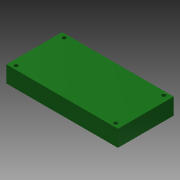
# Autodesk Inventor part: electronics
Saved by Autodesk Inventor 2013 (Build 170138000, 138)
## iProperties
Created: 2013-07-26
Part Number: electronics
Material: Generic
Document SubType Name: Modeling
Designer: employee
Density: 1 g/cm^3
Mass: 25.6248 g
Surface Area: 119.876 cm^2
Volume: 25.6248 cm^3
Author: employee
Autodesk Inventor part; units mm, degrees
ref_plane "YZ Plane" through (0, 0, 0) normal (1, 0, 0) x (0, 1, 0)
ref_plane "XZ Plane" through (0, 0, 0) normal (0, 1, 0) x (-1, 0, 0)
ref_plane "XY Plane" through (0, 0, 0) normal (0, 0, 1) x (1, 0, 0)
sketch "Sketch1" plane through (0, 0, 0) normal (0, 0, 1) x (1, 0, 0)
  line L0 (-50.8, -25.4) -> (50.8, -25.4)
  line L1 (50.8, -25.4) -> (50.8, 25.4)
  line L2 (50.8, 25.4) -> (-50.8, 25.4)
  line L3 (-50.8, 25.4) -> (-50.8, -25.4)
  point P0 (0, 0)
  point P1 (0, 25.4)
  point P2 (50.8, 0)
  dimension "d10" = 6.5
  dimension "d0" = 50.8
  dimension "d2" = 101.6
  constraints: 8 end point, 2 midpoint, 2 parallel, 1 horizontal, 1 horizontal alignment, 1 perpendicular, 1 vertical alignment
  measures "d0" distance of L0.end L1.end
  measures "d2" distance of L0.start L0.end
extrude "Extrusion1" add sketch "Sketch1" along normal blind 15
sketch "Sketch2" plane through (0, 0, 15) normal (0, 0, 1) x (1, 0, 0)
  line L0 (50.8, -25.4) -> (50.8, 25.4) projected
  line L1 (50.8, 25.4) -> (-50.8, 25.4) projected
  line L2 (-45.339, 21.9075) -> (45.339, 21.9075)
  line L3 (45.339, 21.9075) -> (45.339, -21.9075)
  line L4 (45.339, -21.9075) -> (-45.339, -21.9075)
  line L5 (-45.339, -21.9075) -> (-45.339, 21.9075)
  point P0 (45.339, 0)
  point P1 (50.8, 0)
  point P2 (0, 21.9075)
  point P3 (0, 25.4)
  dimension "d5" = 43.815
  dimension "d7" = 90.678
  constraints: 8 end point, 4 midpoint, 2 parallel, 1 horizontal, 1 horizontal alignment, 1 perpendicular, 1 vertical alignment
  measures "d5" distance of L2.end L3.end
  measures "d7" distance of L2.start L2.end
hole "Hole1" at (-45.339, 21.9075, 15) at (45.339, 21.9075, 15) at (45.339, -21.9075, 15) at (-45.339, -21.9075, 15) direction (0, 0, -1) diameter 3.4 end through all clearance for "Socket Head Cap Screw" size "M3" standard "Ansi Metric M Profile"
sketch "Sketch3" plane through (-50.8, -25.4, 0) normal (-1, 0, 0) x (0, 0, 1)
  line L0 (0, 50.8) -> (0, 0) projected
  line L1 (0, 0) -> (15, 0) projected
  circle A0 centre (6, 14.9) radius 5
  point P0 (0, 25.4)
  dimension "d15" = 6
  dimension "d16" = 14.9
  dimension "d17" = 10
  constraints: 1 centre point
  measures "d15" distance from line of A0.centre L0
  measures "d16" distance from line of A0.centre L1
  measures "d17" diameter of A0
extrude "Extrusion2" add sketch "Sketch3" along normal blind 10
sketch "Sketch4" plane through (-50.8, 25.4, 0) normal (-1, 0, 0) x (0, 0, 1)
  circle A0 centre (6, -35.9) radius 5 projected
  line L0 (0, 0) -> (15, 0) projected
  line L1 (-3.5, -12.5) -> (11.5, -12.5)
  line L2 (11.5, -12.5) -> (11.5, -27.5)
  line L3 (11.5, -27.5) -> (-3.5, -27.5)
  line L4 (-3.5, -27.5) -> (-3.5, -12.5)
  point P0 (0, -27.9)
  point P1 (15, -31.5411)
  point P2 (0, -25.4)
  point P3 (-3.5, -20)
  point P4 (4, -12.5)
  dimension "d20" = 20
  dimension "d21" = 15
  dimension "d22" = 15
  dimension "d23" = 2
  constraints: 8 end point, 2 midpoint, 2 parallel, 1 horizontal, 1 perpendicular, 1 other
  measures "d20" distance from line of L0 point (-3.5, -20)
  measures "d21" distance of L3.end L1.start
  measures "d22" distance of L1.start L1.end
  measures "d23" horizontal distance of point (4, -12.5) point (6, -35.9)
extrude "Extrusion3" add sketch "Sketch4" along normal blind 10 contours L1 L2 L3 L4
body "Solid1"
